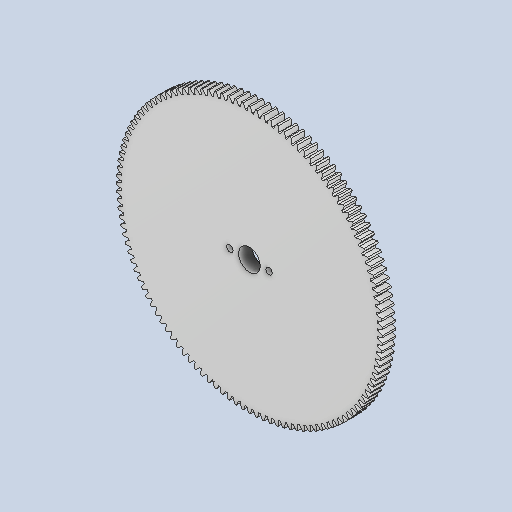
# Autodesk Inventor part: 平歯車1
Saved by Autodesk Inventor 2025.2 (Build 292293000, 293)
## iProperties
CustomPartVersion: 1
Created: 2025-01-13
Part Number: 平歯車1
Material: ABS プラスチック
Document SubType Name: Modeling
Designer: haruy
Categories: <?xml version="1.0" encoding="UTF-16"?> <MemberInstance><Categories><FamilyTemplate><FamilyTemplateParameter ValueType="xs:double" Id="1" ObjectReferenceKey="da_z" ObjectType="kUserParameterObject"/><FamilyTemplateParameter ValueType="xs:double" Id="2" ObjectReferenceKey="da_b" ObjectType="kUserParameterObject"/><FamilyTemplateParameter ValueType="xs:double" Id="3" ObjectReferenceKey="da_beta" ObjectType="kUserParameterObject"/><FamilyTemplateParameter ValueType="xs:double" Id="4" ObjectReferenceKey="da_da" ObjectType="kUserParameterObject"/><FamilyTemplateParameter ValueType="xs:double" Id="5" ObjectReferenceKey="da_aw" ObjectType="kUserParameterObject"/><FamilyTemplateParameter ValueType="xs:string" Id="6" ObjectReferenceKey="EAIAABAAAACIAQAAAAAAAIAAAAAAAAAA" ObjectType="83910656" SubObjectId="SurfaceGeometry"/></FamilyTemplate><ParamToTemplateMap><ParamToTemplate CategoryParameter="//CategoryParameter[@InternalName='046C89C9-8512-4d59-83FE-43B91F4F132A']" TemplateParameter="1"/><ParamToTemplate CategoryParameter="//CategoryParameter[@InternalName='2552DF32-E462-4b46-AEBF-C6C7768E72AC']" TemplateParameter="2"/><ParamToTemplate CategoryParameter="//CategoryParameter[@InternalName='C9EE641D-15FC-4fae-A226-E94C4372FDD7']" TemplateParameter="3"/><ParamToTemplate><ParamToTemplate CategoryParameter="//CategoryParameter[@InternalName='00B6519A-459B-49c7-AD84-2E56D39A5744']" ConstantValue="0.000000"/></ParamToTemplate><ParamToTemplate><ParamToTemplate CategoryParameter="//CategoryParameter[@InternalName='04B31F0E-C7A6-4894-AA32-9629BEFACF47']" ConstantValue="1.000000"/></ParamToTemplate><ParamToTemplate><ParamToTemplate CategoryParameter="//CategoryParameter[@InternalName='43CBEC2E-7847-49e7-A936-2F7889FCB2D9']" ConstantValue="0.250000"/></ParamToTemplate><ParamToTemplate><ParamToTemplate CategoryParameter="//CategoryParameter[@InternalName='B1EFC894-105D-4ebd-86BF-FA20ED196853']" ConstantValue="0.350000"/></ParamToTemplate><ParamToTemplate><ParamToTemplate CategoryParameter="//CategoryParameter[@InternalName='51175063-3D10-4879-93E8-6246FE8B403D']" ConstantValue="2060000000.000000"/></ParamToTemplate><ParamToTemplate><ParamToTemplate CategoryParameter="//CategoryParameter[@InternalName='A3A52E27-4454-46a9-B0BD-C932399B70AF']" ConstantValue="0.300000"/></ParamToTemplate><ParamToTemplate><ParamToTemplate CategoryParameter="//CategoryParameter[@InternalName='91B76062-C214-41d9-B1B9-14D2AB99603D']" ConstantValue="0.100000"/></ParamToTemplate><ParamToTemplate><ParamToTemplate CategoryParameter="//CategoryParameter[@InternalName='374E806E-8B8A-4dda-A9AA-1039D6500AD2']" ConstantValue="10.000000"/></ParamToTemplate><ParamToTemplate><ParamToTemplate CategoryParameter="//CategoryParameter[@InternalName='2D373A89-B862-43d6-8D0B-0CBF12AB9F6C']" ConstantValue="0.349066"/></ParamToTemplate><ParamToTemplate CategoryParameter="//CategoryParameter[@InternalName='37777632-D6A2-4fac-9D53-DB8ACD95C989']" TemplateParameter="4"/><ParamToTemplate CategoryParameter="//CategoryParameter[@InternalName='FD1017F1-B727-4f7e-9707-0F86F1FF9423']" TemplateParameter="5"/><ParamToTemplate><ParamToTemplate CategoryParameter="//CategoryParameter[@InternalName='9E1B4470-B2D3-4ff1-B813-535BB4CDF51A']" ConstantValue="3520000.000000"/></ParamToTemplate><ParamToTemplate><ParamToTemplate CategoryParameter="//CategoryParameter[@InternalName='F8452263-BFF6-458c-9FB1-07C4B99E95CD']" ConstantValue="11400000.000000"/></ParamToTemplate><ParamToTemplate><ParamToTemplate CategoryParameter="//CategoryParameter[@InternalName='3E3BB259-FD49-497f-8171-6EBC954A3479']" ConstantValue="2.000000"/></ParamToTemplate><ParamToTemplate CategoryParameter="//CategoryParameter[@InternalName='27C3BAF2-7550-4e4b-AE2C-0DB134B7D9B7']" TemplateParameter="6"/></ParamToTemplateMap><Category DisplayName="Gear" InternalName="DC85795E-93AB-48d5-8EEE-5A27447B64BD" Mnemonic="Gear"><CategoryParameter DisplayName="z" InternalName="046C89C9-8512-4d59-83FE-43B91F4F132A" Mnemonic="z"/><CategoryParameter DisplayName="b" InternalName="2552DF32-E462-4b46-AEBF-C6C7768E72AC" Mnemonic="b"/><CategoryParameter DisplayName="||b|" InternalName="C9EE641D-15FC-4fae-A226-E94C4372FDD7" Mnemonic="beta"/><CategoryParameter DisplayName="x" InternalName="00B6519A-459B-49c7-AD84-2E56D39A5744" Mnemonic="x"/><CategoryParameter DisplayName="a*" InternalName="04B31F0E-C7A6-4894-AA32-9629BEFACF47" Mnemonic="a"/><CategoryParameter DisplayName="c*" InternalName="43CBEC2E-7847-49e7-A936-2F7889FCB2D9" Mnemonic="c"/><CategoryParameter DisplayName="r|.f|*" InternalName="B1EFC894-105D-4ebd-86BF-FA20ED196853" Mnemonic="rf"/><CategoryParameter DisplayName="E" InternalName="51175063-3D10-4879-93E8-6246FE8B403D" Mnemonic="E"/><CategoryParameter DisplayName="||m|" InternalName="A3A52E27-4454-46a9-B0BD-C932399B70AF" Mnemonic="mi"/><Category DisplayName="SpurGear" InternalName="26C5A22E-A91E-4dfd-A3B3-23CCAFAE1764" Mnemonic="SpurGear"><CategoryParameter DisplayName="m" InternalName="91B76062-C214-41d9-B1B9-14D2AB99603D" Mnemonic="m"/><CategoryParameter DisplayName="P" InternalName="374E806E-8B8A-4dda-A9AA-1039D6500AD2" Mnemonic="PP"/><CategoryParameter DisplayName="||a|" InternalName="2D373A89-B862-43d6-8D0B-0CBF12AB9F6C" Mnemonic="alpha"/><CategoryParameter DisplayName="d|.a|" InternalName="37777632-D6A2-4fac-9D53-DB8ACD95C989" Mnemonic="da"/><CategoryParameter DisplayName="a|.w|" InternalName="FD1017F1-B727-4f7e-9707-0F86F1FF9423" Mnemonic="aw"/><CategoryParameter DisplayName="||s||.Flim|" InternalName="9E1B4470-B2D3-4ff1-B813-535BB4CDF51A" Mnemonic="sFlim"/><CategoryParameter DisplayName="||s||.Hlim|" InternalName="F8452263-BFF6-458c-9FB1-07C4B99E95CD" Mnemonic="sHlim"/><CategoryParameter DisplayName="タイプ" InternalName="3E3BB259-FD49-497f-8171-6EBC954A3479" Mnemonic="type"/><CategoryParameter DisplayName="PitchDiameter" InternalName="27C3BAF2-7550-4e4b-AE2C-0DB134B7D9B7" Mnemonic="IDS_PITCHDIAM"/></Category></Category></Categories></MemberInstance>
Density: 1.06 g/cm^3
Appearance: 滑らか - 白
Mass: 531.343 g
Surface Area: 271.257 cm^2
Volume: 67.687 cm^3
Author: haruy
Autodesk Inventor part; units mm, degrees
sketch "Sketch1" plane through (0, 0, 0) normal (0, 0, 1) x (1, 0, 0)
  circle A0 centre (0, 0) radius 61
  dimension "d0" = 122
  constraints: 1 centre point
  measures "d0" diameter of A0
extrude "Extrusion1" add sketch "Sketch1" along normal blind 6
ref_plane "Work Plane2" through (0, 0, 3) normal (0, 0, 1) x (1, 0, 0)
sketch "Sketch2" plane through (0, 0, 0) normal (0, 0, -1) x (-1, 0, 0)
  circle A0 centre (0, 0) radius 61 projected
  circle A1 centre (0, 0) radius 60
  dimension "d3" = 120
  constraints: 1 centre point, 1 coincident
  measures "d3" diameter of A1
surface extrude "ピッチ円直径" sketch "Sketch2" against normal through all shown no curves A1
ref_plane "Work Plane8" through (0, 0, 0) normal (0.9996573, 0.0261769, 0) x (0, 0, 1)
ref_plane "Work Plane9" through (0, 0, 0) normal (1, 0, 0) x (0, 1, 0)
spur gear teeth "平歯車" teeth 120 pitch diameter 120 tip diameter 122 root diameter 117.5 face width 6 start plane through (0, 0, 0) normal (0, 0, -1) x (-1, 0, 0)
sketch "スケッチ3" plane through (0, 0, 6) normal (0, 0, 1) x (1, 0, 0)
  circle A0 centre (0, 0) radius 5
  circle A1 centre (0, 0) radius 9
  circle A2 centre (-9, 0) radius 1.5
  circle A3 centre (9, 0) radius 1.5
  dimension "d50" = 18
  dimension "d49" = 10
  dimension "d51" = 3
  dimension "d54" = 360
  constraints: 3 centre point, 2 coincident, 1 horizontal alignment, 7 other
  measures "d49" diameter of A0
  measures "d51" diameter of A2
extrude "押し出し2" cut sketch "スケッチ3" against normal blind 10 contours A0 | A1 A3 | A1 A3 | A2 A1 | A1 A2
sketch "スケッチ4" plane through (0, 0, 6) normal (0, 0, 1) x (1, 0, 0)
  circle A0 centre (9, 0) radius 1.5 projected
  circle A1 centre (0, 0) radius 5 projected
  circle A2 centre (-9, 0) radius 1.5 projected
  arc A3 (-3.5911, 60.8942) -> (-4.226, 58.5978) centre (10.0352, 55.8907) ccw projected
  arc A4 (-4.226, 58.5978) -> (-4.9927, 58.5375) centre (0, 0) ccw projected
  arc A5 (-4.9927, 58.5375) -> (-5.979, 60.7063) centre (-18.6549, 53.6328) ccw projected
  arc A6 (-5.979, 60.7063) -> (-6.7732, 60.6228) centre (0, 0) ccw projected
  arc A7 (-6.7732, 60.6228) -> (-7.287, 58.2963) centre (7.0963, 56.3393) ccw projected
  arc A8 (-7.287, 58.2963) -> (-8.0495, 58.1959) centre (0, 0) ccw projected
  arc A9 (-8.0495, 58.1959) -> (-9.148, 60.3102) centre (-21.4362, 52.5829) ccw projected
  arc A10 (-9.148, 60.3102) -> (-9.9366, 60.1852) centre (0, 0) ccw projected
  arc A11 (-9.9366, 60.1852) -> (-10.328, 57.8351) centre (4.138, 56.6335) ccw projected
  arc A12 (-10.328, 57.8351) -> (-11.0842, 57.6949) centre (0, 0) ccw projected
  arc A13 (-11.0842, 57.6949) -> (-12.2918, 59.7487) centre (-24.1588, 51.389) ccw projected
  arc A14 (-12.2918, 59.7487) -> (-13.0729, 59.5827) centre (0, 0) ccw projected
  arc A15 (-13.0729, 59.5827) -> (-13.3407, 57.2153) centre (1.1684, 56.7725) ccw projected
  arc A16 (-13.3407, 57.2153) -> (-14.0885, 57.0357) centre (0, 0) ccw projected
  arc A17 (-14.0885, 57.0357) -> (-15.402, 59.0235) centre (-26.8152, 50.0542) ccw projected
  arc A18 (-15.402, 59.0235) -> (-16.1733, 58.8169) centre (0, 0) ccw projected
  arc A19 (-16.1733, 58.8169) -> (-16.3169, 56.4387) centre (-1.8044, 56.7558) ccw projected
  arc A20 (-16.3169, 56.4387) -> (-17.0542, 56.2202) centre (0, 0) ccw projected
  arc A21 (-17.0542, 56.2202) -> (-18.4699, 58.1366) centre (-29.3981, 48.5822) ccw projected
  arc A22 (-18.4699, 58.1366) -> (-19.2293, 57.8898) centre (0, 0) ccw projected
  arc A23 (-19.2293, 57.8898) -> (-19.2483, 55.5074) centre (-4.7723, 56.5836) ccw projected
  arc A24 (-19.2483, 55.5074) -> (-19.9732, 55.2506) centre (0, 0) ccw projected
  arc A25 (-19.9732, 55.2506) -> (-21.4873, 57.0903) centre (-31.9004, 46.977) ccw projected
  arc A26 (-21.4873, 57.0903) -> (-22.2327, 56.8041) centre (0, 0) ccw projected
  arc A27 (-22.2327, 56.8041) -> (-22.1269, 54.4239) centre (-7.7272, 56.2563) ccw projected
  arc A28 (-22.1269, 54.4239) -> (-22.8374, 54.1296) centre (0, 0) ccw projected
  arc A29 (-22.8374, 54.1296) -> (-24.4457, 55.8875) centre (-34.3153, 45.2431) ccw projected
  arc A30 (-24.4457, 55.8875) -> (-25.1751, 55.5627) centre (0, 0) ccw projected
  arc A31 (-25.1751, 55.5627) -> (-24.9449, 53.1913) centre (-10.6608, 55.7748) ccw projected
  arc A32 (-24.9449, 53.1913) -> (-25.639, 52.8602) centre (0, 0) ccw projected
  arc A33 (-25.639, 52.8602) -> (-27.3371, 54.5315) centre (-36.6361, 43.3852) ccw projected
  arc A34 (-27.3371, 54.5315) -> (-28.0486, 54.169) centre (0, 0) ccw projected
  arc A35 (-28.0486, 54.169) -> (-27.6946, 51.8129) centre (-13.5652, 55.1404) ccw projected
  arc A36 (-27.6946, 51.8129) -> (-28.3704, 51.4459) centre (0, 0) ccw projected
  arc A37 (-28.3704, 51.4459) -> (-30.1536, 53.026) centre (-38.8565, 41.4084) ccw projected
  arc A38 (-30.1536, 53.026) -> (-30.8451, 52.6268) centre (0, 0) ccw projected
  arc A39 (-30.8451, 52.6268) -> (-30.3683, 50.2924) centre (-16.4324, 54.3549) ccw projected
  arc A40 (-30.3683, 50.2924) -> (-31.024, 49.8906) centre (0, 0) ccw projected
  arc A41 (-31.024, 49.8906) -> (-32.8874, 51.3753) centre (-40.9704, 39.318) ccw projected
  arc A42 (-32.8874, 51.3753) -> (-33.5571, 50.9404) centre (0, 0) ccw projected
  arc A43 (-33.5571, 50.9404) -> (-32.9588, 48.6342) centre (-19.2546, 53.4204) ccw projected
  arc A44 (-32.9588, 48.6342) -> (-33.5925, 48.1986) centre (0, 0) ccw projected
  arc A45 (-33.5925, 48.1986) -> (-35.5311, 49.5836) centre (-42.972, 37.1199) ccw projected
  arc A46 (-35.5311, 49.5836) -> (-36.1771, 49.1143) centre (0, 0) ccw projected
  arc A47 (-36.1771, 49.1143) -> (-35.4589, 46.8426) centre (-22.0241, 52.3395) ccw projected
  arc A48 (-35.4589, 46.8426) -> (-36.069, 46.3744) centre (0, 0) ccw projected
  arc A49 (-36.069, 46.3744) -> (-38.0775, 47.6561) centre (-44.8558, 34.8201) ccw projected
  arc A50 (-38.0775, 47.6561) -> (-38.698, 47.1536) centre (0, 0) ccw projected
  arc A51 (-38.698, 47.1536) -> (-37.8619, 44.9226) centre (-24.7331, 51.1151) ccw projected
  arc A52 (-37.8619, 44.9226) -> (-38.4466, 44.4232) centre (0, 0) ccw projected
  arc A53 (-38.4466, 44.4232) -> (-40.5194, 45.598) centre (-46.6167, 32.4248) ccw projected
  arc A54 (-40.5194, 45.598) -> (-41.1128, 45.0637) centre (0, 0) ccw projected
  arc A55 (-41.1128, 45.0637) -> (-40.161, 42.8795) centre (-27.3744, 49.7506) ccw projected
  arc A56 (-40.161, 42.8795) -> (-40.7189, 42.3501) centre (0, 0) ccw projected
  arc A57 (-40.7189, 42.3501) -> (-42.8503, 43.4149) centre (-48.2498, 29.9406) ccw projected
  arc A58 (-42.8503, 43.4149) -> (-43.4149, 42.8503) centre (0, 0) ccw projected
  arc A59 (-43.4149, 42.8503) -> (-42.3501, 40.7189) centre (-29.9406, 48.2498) ccw projected
  arc A60 (-42.3501, 40.7189) -> (-42.8795, 40.161) centre (0, 0) ccw projected
  arc A61 (-42.8795, 40.161) -> (-45.0637, 41.1128) centre (-49.7506, 27.3744) ccw projected
  arc A62 (-45.0637, 41.1128) -> (-45.598, 40.5194) centre (0, 0) ccw projected
  arc A63 (-45.598, 40.5194) -> (-44.4232, 38.4466) centre (-32.4248, 46.6167) ccw projected
  arc A64 (-44.4232, 38.4466) -> (-44.9226, 37.8619) centre (0, 0) ccw projected
  arc A65 (-44.9226, 37.8619) -> (-47.1536, 38.698) centre (-51.1151, 24.7331) ccw projected
  arc A66 (-47.1536, 38.698) -> (-47.6561, 38.0775) centre (0, 0) ccw projected
  arc A67 (-47.6561, 38.0775) -> (-46.3744, 36.069) centre (-34.8201, 44.8558) ccw projected
  arc A68 (-46.3744, 36.069) -> (-46.8426, 35.4589) centre (0, 0) ccw projected
  arc A69 (-46.8426, 35.4589) -> (-49.1143, 36.1771) centre (-52.3395, 22.0241) ccw projected
  arc A70 (-49.1143, 36.1771) -> (-49.5836, 35.5311) centre (0, 0) ccw projected
  arc A71 (-49.5836, 35.5311) -> (-48.1986, 33.5925) centre (-37.1199, 42.972) ccw projected
  arc A72 (-48.1986, 33.5925) -> (-48.6342, 32.9588) centre (0, 0) ccw projected
  arc A73 (-48.6342, 32.9588) -> (-50.9404, 33.5571) centre (-53.4204, 19.2546) ccw projected
  arc A74 (-50.9404, 33.5571) -> (-51.3753, 32.8874) centre (0, 0) ccw projected
  arc A75 (-51.3753, 32.8874) -> (-49.8906, 31.024) centre (-39.318, 40.9704) ccw projected
  arc A76 (-49.8906, 31.024) -> (-50.2924, 30.3683) centre (0, 0) ccw projected
  arc A77 (-50.2924, 30.3683) -> (-52.6268, 30.8451) centre (-54.3549, 16.4324) ccw projected
  arc A78 (-52.6268, 30.8451) -> (-53.026, 30.1536) centre (0, 0) ccw projected
  arc A79 (-53.026, 30.1536) -> (-51.4459, 28.3704) centre (-41.4084, 38.8565) ccw projected
  arc A80 (-51.4459, 28.3704) -> (-51.8129, 27.6946) centre (0, 0) ccw projected
  arc A81 (-51.8129, 27.6946) -> (-54.169, 28.0486) centre (-55.1404, 13.5652) ccw projected
  arc A82 (-54.169, 28.0486) -> (-54.5315, 27.3371) centre (0, 0) ccw projected
  arc A83 (-54.5315, 27.3371) -> (-52.8602, 25.639) centre (-43.3852, 36.6361) ccw projected
  arc A84 (-52.8602, 25.639) -> (-53.1913, 24.9449) centre (0, 0) ccw projected
  arc A85 (-53.1913, 24.9449) -> (-55.5627, 25.1751) centre (-55.7748, 10.6608) ccw projected
  arc A86 (-55.5627, 25.1751) -> (-55.8875, 24.4457) centre (0, 0) ccw projected
  arc A87 (-55.8875, 24.4457) -> (-54.1296, 22.8374) centre (-45.2431, 34.3153) ccw projected
  arc A88 (-54.1296, 22.8374) -> (-54.4239, 22.1269) centre (0, 0) ccw projected
  arc A89 (-54.4239, 22.1269) -> (-56.8041, 22.2327) centre (-56.2563, 7.7272) ccw projected
  arc A90 (-56.8041, 22.2327) -> (-57.0903, 21.4873) centre (0, 0) ccw projected
  arc A91 (-57.0903, 21.4873) -> (-55.2506, 19.9732) centre (-46.977, 31.9004) ccw projected
  arc A92 (-55.2506, 19.9732) -> (-55.5074, 19.2483) centre (0, 0) ccw projected
  arc A93 (-55.5074, 19.2483) -> (-57.8898, 19.2293) centre (-56.5836, 4.7723) ccw projected
  arc A94 (-57.8898, 19.2293) -> (-58.1366, 18.4699) centre (0, 0) ccw projected
  arc A95 (-58.1366, 18.4699) -> (-56.2202, 17.0542) centre (-48.5822, 29.3981) ccw projected
  arc A96 (-56.2202, 17.0542) -> (-56.4387, 16.3169) centre (0, 0) ccw projected
  arc A97 (-56.4387, 16.3169) -> (-58.8169, 16.1733) centre (-56.7558, 1.8044) ccw projected
  arc A98 (-58.8169, 16.1733) -> (-59.0235, 15.402) centre (0, 0) ccw projected
  arc A99 (-59.0235, 15.402) -> (-57.0357, 14.0885) centre (-50.0542, 26.8152) ccw projected
  arc A100 (-57.0357, 14.0885) -> (-57.2153, 13.3407) centre (0, 0) ccw projected
  arc A101 (-57.2153, 13.3407) -> (-59.5827, 13.0729) centre (-56.7725, -1.1684) ccw projected
  arc A102 (-59.5827, 13.0729) -> (-59.7487, 12.2918) centre (0, 0) ccw projected
  arc A103 (-59.7487, 12.2918) -> (-57.6949, 11.0842) centre (-51.389, 24.1588) ccw projected
  arc A104 (-57.6949, 11.0842) -> (-57.8351, 10.328) centre (0, 0) ccw projected
  arc A105 (-57.8351, 10.328) -> (-60.1852, 9.9366) centre (-56.6335, -4.138) ccw projected
  arc A106 (-60.1852, 9.9366) -> (-60.3102, 9.148) centre (0, 0) ccw projected
  arc A107 (-60.3102, 9.148) -> (-58.1959, 8.0495) centre (-52.5829, 21.4362) ccw projected
  arc A108 (-58.1959, 8.0495) -> (-58.2963, 7.287) centre (0, 0) ccw projected
  arc A109 (-58.2963, 7.287) -> (-60.6228, 6.7732) centre (-56.3393, -7.0963) ccw projected
  arc A110 (-60.6228, 6.7732) -> (-60.7063, 5.979) centre (0, 0) ccw projected
  arc A111 (-60.7063, 5.979) -> (-58.5375, 4.9927) centre (-53.6328, 18.6549) ccw projected
  arc A112 (-58.5375, 4.9927) -> (-58.5978, 4.226) centre (0, 0) ccw projected
  arc A113 (-58.5978, 4.226) -> (-60.8942, 3.5911) centre (-55.8907, -10.0352) ccw projected
  arc A114 (-60.8942, 3.5911) -> (-60.936, 2.7937) centre (0, 0) ccw projected
  arc A115 (-60.936, 2.7937) -> (-58.7185, 1.9222) centre (-54.5356, 15.8224) ccw projected
  arc A116 (-58.7185, 1.9222) -> (-58.7387, 1.1535) centre (0, 0) ccw projected
  arc A117 (-58.7387, 1.1535) -> (-60.9987, 0.3992) centre (-55.2889, -12.9465) ccw projected
  arc A118 (-60.9987, 0.3992) -> (-60.9987, -0.3992) centre (0, 0) ccw projected
  arc A119 (-60.9987, -0.3992) -> (-58.7387, -1.1535) centre (-55.2889, 12.9465) ccw projected
  arc A120 (-58.7387, -1.1535) -> (-58.7185, -1.9222) centre (0, 0) ccw projected
  arc A121 (-58.7185, -1.9222) -> (-60.936, -2.7937) centre (-54.5356, -15.8224) ccw projected
  arc A122 (-60.936, -2.7937) -> (-60.8942, -3.5911) centre (0, 0) ccw projected
  arc A123 (-60.8942, -3.5911) -> (-58.5978, -4.226) centre (-55.8907, 10.0352) ccw projected
  arc A124 (-58.5978, -4.226) -> (-58.5375, -4.9927) centre (0, 0) ccw projected
  arc A125 (-58.5375, -4.9927) -> (-60.7063, -5.979) centre (-53.6328, -18.6549) ccw projected
  arc A126 (-60.7063, -5.979) -> (-60.6228, -6.7732) centre (0, 0) ccw projected
  arc A127 (-60.6228, -6.7732) -> (-58.2963, -7.287) centre (-56.3393, 7.0963) ccw projected
  arc A128 (-58.2963, -7.287) -> (-58.1959, -8.0495) centre (0, 0) ccw projected
  arc A129 (-58.1959, -8.0495) -> (-60.3102, -9.148) centre (-52.5829, -21.4362) ccw projected
  arc A130 (-60.3102, -9.148) -> (-60.1852, -9.9366) centre (0, 0) ccw projected
  arc A131 (-60.1852, -9.9366) -> (-57.8351, -10.328) centre (-56.6335, 4.138) ccw projected
  arc A132 (-57.8351, -10.328) -> (-57.6949, -11.0842) centre (0, 0) ccw projected
  arc A133 (-57.6949, -11.0842) -> (-59.7487, -12.2918) centre (-51.389, -24.1588) ccw projected
  arc A134 (-59.7487, -12.2918) -> (-59.5827, -13.0729) centre (0, 0) ccw projected
  arc A135 (-59.5827, -13.0729) -> (-57.2153, -13.3407) centre (-56.7725, 1.1684) ccw projected
  arc A136 (-57.2153, -13.3407) -> (-57.0357, -14.0885) centre (0, 0) ccw projected
  arc A137 (-57.0357, -14.0885) -> (-59.0235, -15.402) centre (-50.0542, -26.8152) ccw projected
  arc A138 (-59.0235, -15.402) -> (-58.8169, -16.1733) centre (0, 0) ccw projected
  arc A139 (-58.8169, -16.1733) -> (-56.4387, -16.3169) centre (-56.7558, -1.8044) ccw projected
  arc A140 (-56.4387, -16.3169) -> (-56.2202, -17.0542) centre (0, 0) ccw projected
  arc A141 (-56.2202, -17.0542) -> (-58.1366, -18.4699) centre (-48.5822, -29.3981) ccw projected
  arc A142 (-58.1366, -18.4699) -> (-57.8898, -19.2293) centre (0, 0) ccw projected
  arc A143 (-57.8898, -19.2293) -> (-55.5074, -19.2483) centre (-56.5836, -4.7723) ccw projected
  arc A144 (-55.5074, -19.2483) -> (-55.2506, -19.9732) centre (0, 0) ccw projected
  arc A145 (-55.2506, -19.9732) -> (-57.0903, -21.4873) centre (-46.977, -31.9004) ccw projected
  arc A146 (-57.0903, -21.4873) -> (-56.8041, -22.2327) centre (0, 0) ccw projected
  arc A147 (-56.8041, -22.2327) -> (-54.4239, -22.1269) centre (-56.2563, -7.7272) ccw projected
  arc A148 (-54.4239, -22.1269) -> (-54.1296, -22.8374) centre (0, 0) ccw projected
  arc A149 (-54.1296, -22.8374) -> (-55.8875, -24.4457) centre (-45.2431, -34.3153) ccw projected
  arc A150 (-55.8875, -24.4457) -> (-55.5627, -25.1751) centre (0, 0) ccw projected
  arc A151 (-55.5627, -25.1751) -> (-53.1913, -24.9449) centre (-55.7748, -10.6608) ccw projected
  arc A152 (-53.1913, -24.9449) -> (-52.8602, -25.639) centre (0, 0) ccw projected
  arc A153 (-52.8602, -25.639) -> (-54.5315, -27.3371) centre (-43.3852, -36.6361) ccw projected
  arc A154 (-54.5315, -27.3371) -> (-54.169, -28.0486) centre (0, 0) ccw projected
  arc A155 (-54.169, -28.0486) -> (-51.8129, -27.6946) centre (-55.1404, -13.5652) ccw projected
  arc A156 (-51.8129, -27.6946) -> (-51.4459, -28.3704) centre (0, 0) ccw projected
  arc A157 (-51.4459, -28.3704) -> (-53.026, -30.1536) centre (-41.4084, -38.8565) ccw projected
  arc A158 (-53.026, -30.1536) -> (-52.6268, -30.8451) centre (0, 0) ccw projected
  arc A159 (-52.6268, -30.8451) -> (-50.2924, -30.3683) centre (-54.3549, -16.4324) ccw projected
  arc A160 (-50.2924, -30.3683) -> (-49.8906, -31.024) centre (0, 0) ccw projected
  arc A161 (-49.8906, -31.024) -> (-51.3753, -32.8874) centre (-39.318, -40.9704) ccw projected
  arc A162 (-51.3753, -32.8874) -> (-50.9404, -33.5571) centre (0, 0) ccw projected
  arc A163 (-50.9404, -33.5571) -> (-48.6342, -32.9588) centre (-53.4204, -19.2546) ccw projected
  arc A164 (-48.6342, -32.9588) -> (-48.1986, -33.5925) centre (0, 0) ccw projected
  arc A165 (-48.1986, -33.5925) -> (-49.5836, -35.5311) centre (-37.1199, -42.972) ccw projected
  arc A166 (-49.5836, -35.5311) -> (-49.1143, -36.1771) centre (0, 0) ccw projected
  arc A167 (-49.1143, -36.1771) -> (-46.8426, -35.4589) centre (-52.3395, -22.0241) ccw projected
  arc A168 (-46.8426, -35.4589) -> (-46.3744, -36.069) centre (0, 0) ccw projected
  arc A169 (-46.3744, -36.069) -> (-47.6561, -38.0775) centre (-34.8201, -44.8558) ccw projected
  arc A170 (-47.6561, -38.0775) -> (-47.1536, -38.698) centre (0, 0) ccw projected
  arc A171 (-47.1536, -38.698) -> (-44.9226, -37.8619) centre (-51.1151, -24.7331) ccw projected
  arc A172 (-44.9226, -37.8619) -> (-44.4232, -38.4466) centre (0, 0) ccw projected
  arc A173 (-44.4232, -38.4466) -> (-45.598, -40.5194) centre (-32.4248, -46.6167) ccw projected
  arc A174 (-45.598, -40.5194) -> (-45.0637, -41.1128) centre (0, 0) ccw projected
  arc A175 (-45.0637, -41.1128) -> (-42.8795, -40.161) centre (-49.7506, -27.3744) ccw projected
  arc A176 (-42.8795, -40.161) -> (-42.3501, -40.7189) centre (0, 0) ccw projected
  arc A177 (-42.3501, -40.7189) -> (-43.4149, -42.8503) centre (-29.9406, -48.2498) ccw projected
  arc A178 (-43.4149, -42.8503) -> (-42.8503, -43.4149) centre (0, 0) ccw projected
  arc A179 (-42.8503, -43.4149) -> (-40.7189, -42.3501) centre (-48.2498, -29.9406) ccw projected
  arc A180 (-40.7189, -42.3501) -> (-40.161, -42.8795) centre (0, 0) ccw projected
  arc A181 (-40.161, -42.8795) -> (-41.1128, -45.0637) centre (-27.3744, -49.7506) ccw projected
  arc A182 (-41.1128, -45.0637) -> (-40.5194, -45.598) centre (0, 0) ccw projected
  arc A183 (-40.5194, -45.598) -> (-38.4466, -44.4232) centre (-46.6167, -32.4248) ccw projected
  arc A184 (-38.4466, -44.4232) -> (-37.8619, -44.9226) centre (0, 0) ccw projected
  arc A185 (-37.8619, -44.9226) -> (-38.698, -47.1536) centre (-24.7331, -51.1151) ccw projected
  arc A186 (-38.698, -47.1536) -> (-38.0775, -47.6561) centre (0, 0) ccw projected
  arc A187 (-38.0775, -47.6561) -> (-36.069, -46.3744) centre (-44.8558, -34.8201) ccw projected
  arc A188 (-36.069, -46.3744) -> (-35.4589, -46.8426) centre (0, 0) ccw projected
  arc A189 (-35.4589, -46.8426) -> (-36.1771, -49.1143) centre (-22.0241, -52.3395) ccw projected
  arc A190 (-36.1771, -49.1143) -> (-35.5311, -49.5836) centre (0, 0) ccw projected
  arc A191 (-35.5311, -49.5836) -> (-33.5925, -48.1986) centre (-42.972, -37.1199) ccw projected
  arc A192 (-33.5925, -48.1986) -> (-32.9588, -48.6342) centre (0, 0) ccw projected
  arc A193 (-32.9588, -48.6342) -> (-33.5571, -50.9404) centre (-19.2546, -53.4204) ccw projected
  arc A194 (-33.5571, -50.9404) -> (-32.8874, -51.3753) centre (0, 0) ccw projected
  arc A195 (-32.8874, -51.3753) -> (-31.024, -49.8906) centre (-40.9704, -39.318) ccw projected
  arc A196 (-31.024, -49.8906) -> (-30.3683, -50.2924) centre (0, 0) ccw projected
  arc A197 (-30.3683, -50.2924) -> (-30.8451, -52.6268) centre (-16.4324, -54.3549) ccw projected
  arc A198 (-30.8451, -52.6268) -> (-30.1536, -53.026) centre (0, 0) ccw projected
  arc A199 (-30.1536, -53.026) -> (-28.3704, -51.4459) centre (-38.8565, -41.4084) ccw projected
  arc A200 (-28.3704, -51.4459) -> (-27.6946, -51.8129) centre (0, 0) ccw projected
  arc A201 (-27.6946, -51.8129) -> (-28.0486, -54.169) centre (-13.5652, -55.1404) ccw projected
  arc A202 (-28.0486, -54.169) -> (-27.3371, -54.5315) centre (0, 0) ccw projected
  arc A203 (-27.3371, -54.5315) -> (-25.639, -52.8602) centre (-36.6361, -43.3852) ccw projected
  arc A204 (-25.639, -52.8602) -> (-24.9449, -53.1913) centre (0, 0) ccw projected
  arc A205 (-24.9449, -53.1913) -> (-25.1751, -55.5627) centre (-10.6608, -55.7748) ccw projected
  arc A206 (-25.1751, -55.5627) -> (-24.4457, -55.8875) centre (0, 0) ccw projected
  arc A207 (-24.4457, -55.8875) -> (-22.8374, -54.1296) centre (-34.3153, -45.2431) ccw projected
  arc A208 (-22.8374, -54.1296) -> (-22.1269, -54.4239) centre (0, 0) ccw projected
  arc A209 (-22.1269, -54.4239) -> (-22.2327, -56.8041) centre (-7.7272, -56.2563) ccw projected
  arc A210 (-22.2327, -56.8041) -> (-21.4873, -57.0903) centre (0, 0) ccw projected
  arc A211 (-21.4873, -57.0903) -> (-19.9732, -55.2506) centre (-31.9004, -46.977) ccw projected
  arc A212 (-19.9732, -55.2506) -> (-19.2483, -55.5074) centre (0, 0) ccw projected
  arc A213 (-19.2483, -55.5074) -> (-19.2293, -57.8898) centre (-4.7723, -56.5836) ccw projected
  arc A214 (-19.2293, -57.8898) -> (-18.4699, -58.1366) centre (0, 0) ccw projected
  arc A215 (-18.4699, -58.1366) -> (-17.0542, -56.2202) centre (-29.3981, -48.5822) ccw projected
  arc A216 (-17.0542, -56.2202) -> (-16.3169, -56.4387) centre (0, 0) ccw projected
  arc A217 (-16.3169, -56.4387) -> (-16.1733, -58.8169) centre (-1.8044, -56.7558) ccw projected
  arc A218 (-16.1733, -58.8169) -> (-15.402, -59.0235) centre (0, 0) ccw projected
  arc A219 (-15.402, -59.0235) -> (-14.0885, -57.0357) centre (-26.8152, -50.0542) ccw projected
  arc A220 (-14.0885, -57.0357) -> (-13.3407, -57.2153) centre (0, 0) ccw projected
  arc A221 (-13.3407, -57.2153) -> (-13.0729, -59.5827) centre (1.1684, -56.7725) ccw projected
  arc A222 (-13.0729, -59.5827) -> (-12.2918, -59.7487) centre (0, 0) ccw projected
  arc A223 (-12.2918, -59.7487) -> (-11.0842, -57.6949) centre (-24.1588, -51.389) ccw projected
  arc A224 (-11.0842, -57.6949) -> (-10.328, -57.8351) centre (0, 0) ccw projected
  arc A225 (-10.328, -57.8351) -> (-9.9366, -60.1852) centre (4.138, -56.6335) ccw projected
  arc A226 (-9.9366, -60.1852) -> (-9.148, -60.3102) centre (0, 0) ccw projected
  arc A227 (-9.148, -60.3102) -> (-8.0495, -58.1959) centre (-21.4362, -52.5829) ccw projected
  arc A228 (-8.0495, -58.1959) -> (-7.287, -58.2963) centre (0, 0) ccw projected
  arc A229 (-7.287, -58.2963) -> (-6.7732, -60.6228) centre (7.0963, -56.3393) ccw projected
  arc A230 (-6.7732, -60.6228) -> (-5.979, -60.7063) centre (0, 0) ccw projected
  arc A231 (-5.979, -60.7063) -> (-4.9927, -58.5375) centre (-18.6549, -53.6328) ccw projected
  arc A232 (-4.9927, -58.5375) -> (-4.226, -58.5978) centre (0, 0) ccw projected
  arc A233 (-4.226, -58.5978) -> (-3.5911, -60.8942) centre (10.0352, -55.8907) ccw projected
  arc A234 (-3.5911, -60.8942) -> (-2.7937, -60.936) centre (0, 0) ccw projected
  arc A235 (-2.7937, -60.936) -> (-1.9222, -58.7185) centre (-15.8224, -54.5356) ccw projected
  arc A236 (-1.9222, -58.7185) -> (-1.1535, -58.7387) centre (0, 0) ccw projected
  arc A237 (-1.1535, -58.7387) -> (-0.3992, -60.9987) centre (12.9465, -55.2889) ccw projected
  arc A238 (-0.3992, -60.9987) -> (0.3992, -60.9987) centre (0, 0) ccw projected
  arc A239 (0.3992, -60.9987) -> (1.1535, -58.7387) centre (-12.9465, -55.2889) ccw projected
  arc A240 (1.1535, -58.7387) -> (1.9222, -58.7185) centre (0, 0) ccw projected
  arc A241 (1.9222, -58.7185) -> (2.7937, -60.936) centre (15.8224, -54.5356) ccw projected
  arc A242 (2.7937, -60.936) -> (3.5911, -60.8942) centre (0, 0) ccw projected
  arc A243 (3.5911, -60.8942) -> (4.226, -58.5978) centre (-10.0352, -55.8907) ccw projected
  arc A244 (4.226, -58.5978) -> (4.9927, -58.5375) centre (0, 0) ccw projected
  arc A245 (4.9927, -58.5375) -> (5.979, -60.7063) centre (18.6549, -53.6328) ccw projected
  arc A246 (5.979, -60.7063) -> (6.7732, -60.6228) centre (0, 0) ccw projected
  arc A247 (6.7732, -60.6228) -> (7.287, -58.2963) centre (-7.0963, -56.3393) ccw projected
  arc A248 (7.287, -58.2963) -> (8.0495, -58.1959) centre (0, 0) ccw projected
  arc A249 (8.0495, -58.1959) -> (9.148, -60.3102) centre (21.4362, -52.5829) ccw projected
  arc A250 (9.148, -60.3102) -> (9.9366, -60.1852) centre (0, 0) ccw projected
  arc A251 (9.9366, -60.1852) -> (10.328, -57.8351) centre (-4.138, -56.6335) ccw projected
  arc A252 (10.328, -57.8351) -> (11.0842, -57.6949) centre (0, 0) ccw projected
  arc A253 (11.0842, -57.6949) -> (12.2918, -59.7487) centre (24.1588, -51.389) ccw projected
  arc A254 (12.2918, -59.7487) -> (13.0729, -59.5827) centre (0, 0) ccw projected
  arc A255 (13.0729, -59.5827) -> (13.3407, -57.2153) centre (-1.1684, -56.7725) ccw projected
  arc A256 (13.3407, -57.2153) -> (14.0885, -57.0357) centre (0, 0) ccw projected
  arc A257 (14.0885, -57.0357) -> (15.402, -59.0235) centre (26.8152, -50.0542) ccw projected
  arc A258 (15.402, -59.0235) -> (16.1733, -58.8169) centre (0, 0) ccw projected
  arc A259 (16.1733, -58.8169) -> (16.3169, -56.4387) centre (1.8044, -56.7558) ccw projected
  arc A260 (16.3169, -56.4387) -> (17.0542, -56.2202) centre (0, 0) ccw projected
  arc A261 (17.0542, -56.2202) -> (18.4699, -58.1366) centre (29.3981, -48.5822) ccw projected
  arc A262 (18.4699, -58.1366) -> (19.2293, -57.8898) centre (0, 0) ccw projected
  arc A263 (19.2293, -57.8898) -> (19.2483, -55.5074) centre (4.7723, -56.5836) ccw projected
  arc A264 (19.2483, -55.5074) -> (19.9732, -55.2506) centre (0, 0) ccw projected
  arc A265 (19.9732, -55.2506) -> (21.4873, -57.0903) centre (31.9004, -46.977) ccw projected
  arc A266 (21.4873, -57.0903) -> (22.2327, -56.8041) centre (0, 0) ccw projected
  arc A267 (22.2327, -56.8041) -> (22.1269, -54.4239) centre (7.7272, -56.2563) ccw projected
  arc A268 (22.1269, -54.4239) -> (22.8374, -54.1296) centre (0, 0) ccw projected
  arc A269 (22.8374, -54.1296) -> (24.4457, -55.8875) centre (34.3153, -45.2431) ccw projected
  arc A270 (24.4457, -55.8875) -> (25.1751, -55.5627) centre (0, 0) ccw projected
  arc A271 (25.1751, -55.5627) -> (24.9449, -53.1913) centre (10.6608, -55.7748) ccw projected
  arc A272 (24.9449, -53.1913) -> (25.639, -52.8602) centre (0, 0) ccw projected
  arc A273 (25.639, -52.8602) -> (27.3371, -54.5315) centre (36.6361, -43.3852) ccw projected
  arc A274 (27.3371, -54.5315) -> (28.0486, -54.169) centre (0, 0) ccw projected
  arc A275 (28.0486, -54.169) -> (27.6946, -51.8129) centre (13.5652, -55.1404) ccw projected
  arc A276 (27.6946, -51.8129) -> (28.3704, -51.4459) centre (0, 0) ccw projected
  arc A277 (28.3704, -51.4459) -> (30.1536, -53.026) centre (38.8565, -41.4084) ccw projected
  arc A278 (30.1536, -53.026) -> (30.8451, -52.6268) centre (0, 0) ccw projected
  arc A279 (30.8451, -52.6268) -> (30.3683, -50.2924) centre (16.4324, -54.3549) ccw projected
  arc A280 (30.3683, -50.2924) -> (31.024, -49.8906) centre (0, 0) ccw projected
  arc A281 (31.024, -49.8906) -> (32.8874, -51.3753) centre (40.9704, -39.318) ccw projected
  arc A282 (32.8874, -51.3753) -> (33.5571, -50.9404) centre (0, 0) ccw projected
  arc A283 (33.5571, -50.9404) -> (32.9588, -48.6342) centre (19.2546, -53.4204) ccw projected
  arc A284 (32.9588, -48.6342) -> (33.5925, -48.1986) centre (0, 0) ccw projected
  arc A285 (33.5925, -48.1986) -> (35.5311, -49.5836) centre (42.972, -37.1199) ccw projected
  arc A286 (35.5311, -49.5836) -> (36.1771, -49.1143) centre (0, 0) ccw projected
  arc A287 (36.1771, -49.1143) -> (35.4589, -46.8426) centre (22.0241, -52.3395) ccw projected
  arc A288 (35.4589, -46.8426) -> (36.069, -46.3744) centre (0, 0) ccw projected
  arc A289 (36.069, -46.3744) -> (38.0775, -47.6561) centre (44.8558, -34.8201) ccw projected
  arc A290 (38.0775, -47.6561) -> (38.698, -47.1536) centre (0, 0) ccw projected
  arc A291 (38.698, -47.1536) -> (37.8619, -44.9226) centre (24.7331, -51.1151) ccw projected
  arc A292 (37.8619, -44.9226) -> (38.4466, -44.4232) centre (0, 0) ccw projected
  arc A293 (38.4466, -44.4232) -> (40.5194, -45.598) centre (46.6167, -32.4248) ccw projected
  arc A294 (40.5194, -45.598) -> (41.1128, -45.0637) centre (0, 0) ccw projected
  arc A295 (41.1128, -45.0637) -> (40.161, -42.8795) centre (27.3744, -49.7506) ccw projected
  arc A296 (40.161, -42.8795) -> (40.7189, -42.3501) centre (0, 0) ccw projected
  arc A297 (40.7189, -42.3501) -> (42.8503, -43.4149) centre (48.2498, -29.9406) ccw projected
  arc A298 (42.8503, -43.4149) -> (43.4149, -42.8503) centre (0, 0) ccw projected
  arc A299 (43.4149, -42.8503) -> (42.3501, -40.7189) centre (29.9406, -48.2498) ccw projected
  arc A300 (42.3501, -40.7189) -> (42.8795, -40.161) centre (0, 0) ccw projected
  arc A301 (42.8795, -40.161) -> (45.0637, -41.1128) centre (49.7506, -27.3744) ccw projected
  arc A302 (45.0637, -41.1128) -> (45.598, -40.5194) centre (0, 0) ccw projected
  arc A303 (45.598, -40.5194) -> (44.4232, -38.4466) centre (32.4248, -46.6167) ccw projected
  arc A304 (44.4232, -38.4466) -> (44.9226, -37.8619) centre (0, 0) ccw projected
  arc A305 (44.9226, -37.8619) -> (47.1536, -38.698) centre (51.1151, -24.7331) ccw projected
  arc A306 (47.1536, -38.698) -> (47.6561, -38.0775) centre (0, 0) ccw projected
  arc A307 (47.6561, -38.0775) -> (46.3744, -36.069) centre (34.8201, -44.8558) ccw projected
  arc A308 (46.3744, -36.069) -> (46.8426, -35.4589) centre (0, 0) ccw projected
  arc A309 (46.8426, -35.4589) -> (49.1143, -36.1771) centre (52.3395, -22.0241) ccw projected
  arc A310 (49.1143, -36.1771) -> (49.5836, -35.5311) centre (0, 0) ccw projected
  arc A311 (49.5836, -35.5311) -> (48.1986, -33.5925) centre (37.1199, -42.972) ccw projected
  arc A312 (48.1986, -33.5925) -> (48.6342, -32.9588) centre (0, 0) ccw projected
  arc A313 (48.6342, -32.9588) -> (50.9404, -33.5571) centre (53.4204, -19.2546) ccw projected
  arc A314 (50.9404, -33.5571) -> (51.3753, -32.8874) centre (0, 0) ccw projected
  arc A315 (51.3753, -32.8874) -> (49.8906, -31.024) centre (39.318, -40.9704) ccw projected
  arc A316 (49.8906, -31.024) -> (50.2924, -30.3683) centre (0, 0) ccw projected
  arc A317 (50.2924, -30.3683) -> (52.6268, -30.8451) centre (54.3549, -16.4324) ccw projected
  arc A318 (52.6268, -30.8451) -> (53.026, -30.1536) centre (0, 0) ccw projected
  arc A319 (53.026, -30.1536) -> (51.4459, -28.3704) centre (41.4084, -38.8565) ccw projected
  arc A320 (51.4459, -28.3704) -> (51.8129, -27.6946) centre (0, 0) ccw projected
  arc A321 (51.8129, -27.6946) -> (54.169, -28.0486) centre (55.1404, -13.5652) ccw projected
  arc A322 (54.169, -28.0486) -> (54.5315, -27.3371) centre (0, 0) ccw projected
  arc A323 (54.5315, -27.3371) -> (52.8602, -25.639) centre (43.3852, -36.6361) ccw projected
  arc A324 (52.8602, -25.639) -> (53.1913, -24.9449) centre (0, 0) ccw projected
  arc A325 (53.1913, -24.9449) -> (55.5627, -25.1751) centre (55.7748, -10.6608) ccw projected
  arc A326 (55.5627, -25.1751) -> (55.8875, -24.4457) centre (0, 0) ccw projected
  arc A327 (55.8875, -24.4457) -> (54.1296, -22.8374) centre (45.2431, -34.3153) ccw projected
  arc A328 (54.1296, -22.8374) -> (54.4239, -22.1269) centre (0, 0) ccw projected
  arc A329 (54.4239, -22.1269) -> (56.8041, -22.2327) centre (56.2563, -7.7272) ccw projected
  arc A330 (56.8041, -22.2327) -> (57.0903, -21.4873) centre (0, 0) ccw projected
  arc A331 (57.0903, -21.4873) -> (55.2506, -19.9732) centre (46.977, -31.9004) ccw projected
  arc A332 (55.2506, -19.9732) -> (55.5074, -19.2483) centre (0, 0) ccw projected
  arc A333 (55.5074, -19.2483) -> (57.8898, -19.2293) centre (56.5836, -4.7723) ccw projected
  arc A334 (57.8898, -19.2293) -> (58.1366, -18.4699) centre (0, 0) ccw projected
  arc A335 (58.1366, -18.4699) -> (56.2202, -17.0542) centre (48.5822, -29.3981) ccw projected
  arc A336 (56.2202, -17.0542) -> (56.4387, -16.3169) centre (0, 0) ccw projected
  arc A337 (56.4387, -16.3169) -> (58.8169, -16.1733) centre (56.7558, -1.8044) ccw projected
  arc A338 (58.8169, -16.1733) -> (59.0235, -15.402) centre (0, 0) ccw projected
  arc A339 (59.0235, -15.402) -> (57.0357, -14.0885) centre (50.0542, -26.8152) ccw projected
  arc A340 (57.0357, -14.0885) -> (57.2153, -13.3407) centre (0, 0) ccw projected
  arc A341 (57.2153, -13.3407) -> (59.5827, -13.0729) centre (56.7725, 1.1684) ccw projected
  arc A342 (59.5827, -13.0729) -> (59.7487, -12.2918) centre (0, 0) ccw projected
  arc A343 (59.7487, -12.2918) -> (57.6949, -11.0842) centre (51.389, -24.1588) ccw projected
  arc A344 (57.6949, -11.0842) -> (57.8351, -10.328) centre (0, 0) ccw projected
  arc A345 (57.8351, -10.328) -> (60.1852, -9.9366) centre (56.6335, 4.138) ccw projected
  arc A346 (60.1852, -9.9366) -> (60.3102, -9.148) centre (0, 0) ccw projected
  arc A347 (60.3102, -9.148) -> (58.1959, -8.0495) centre (52.5829, -21.4362) ccw projected
  arc A348 (58.1959, -8.0495) -> (58.2963, -7.287) centre (0, 0) ccw projected
  arc A349 (58.2963, -7.287) -> (60.6228, -6.7732) centre (56.3393, 7.0963) ccw projected
  arc A350 (60.6228, -6.7732) -> (60.7063, -5.979) centre (0, 0) ccw projected
  arc A351 (60.7063, -5.979) -> (58.5375, -4.9927) centre (53.6328, -18.6549) ccw projected
  arc A352 (58.5375, -4.9927) -> (58.5978, -4.226) centre (0, 0) ccw projected
  arc A353 (58.5978, -4.226) -> (60.8942, -3.5911) centre (55.8907, 10.0352) ccw projected
  arc A354 (60.8942, -3.5911) -> (60.936, -2.7937) centre (0, 0) ccw projected
  arc A355 (60.936, -2.7937) -> (58.7185, -1.9222) centre (54.5356, -15.8224) ccw projected
  arc A356 (58.7185, -1.9222) -> (58.7387, -1.1535) centre (0, 0) ccw projected
  arc A357 (58.7387, -1.1535) -> (60.9987, -0.3992) centre (55.2889, 12.9465) ccw projected
  arc A358 (60.9987, -0.3992) -> (60.9987, 0.3992) centre (0, 0) ccw projected
  arc A359 (60.9987, 0.3992) -> (58.7387, 1.1535) centre (55.2889, -12.9465) ccw projected
  arc A360 (58.7387, 1.1535) -> (58.7185, 1.9222) centre (0, 0) ccw projected
  arc A361 (58.7185, 1.9222) -> (60.936, 2.7937) centre (54.5356, 15.8224) ccw projected
  arc A362 (60.936, 2.7937) -> (60.8942, 3.5911) centre (0, 0) ccw projected
  arc A363 (60.8942, 3.5911) -> (58.5978, 4.226) centre (55.8907, -10.0352) ccw projected
  arc A364 (58.5978, 4.226) -> (58.5375, 4.9927) centre (0, 0) ccw projected
  arc A365 (58.5375, 4.9927) -> (60.7063, 5.979) centre (53.6328, 18.6549) ccw projected
  arc A366 (60.7063, 5.979) -> (60.6228, 6.7732) centre (0, 0) ccw projected
  arc A367 (60.6228, 6.7732) -> (58.2963, 7.287) centre (56.3393, -7.0963) ccw projected
  arc A368 (58.2963, 7.287) -> (58.1959, 8.0495) centre (0, 0) ccw projected
  arc A369 (58.1959, 8.0495) -> (60.3102, 9.148) centre (52.5829, 21.4362) ccw projected
  arc A370 (60.3102, 9.148) -> (60.1852, 9.9366) centre (0, 0) ccw projected
  arc A371 (60.1852, 9.9366) -> (57.8351, 10.328) centre (56.6335, -4.138) ccw projected
  arc A372 (57.8351, 10.328) -> (57.6949, 11.0842) centre (0, 0) ccw projected
  arc A373 (57.6949, 11.0842) -> (59.7487, 12.2918) centre (51.389, 24.1588) ccw projected
  arc A374 (59.7487, 12.2918) -> (59.5827, 13.0729) centre (0, 0) ccw projected
  arc A375 (59.5827, 13.0729) -> (57.2153, 13.3407) centre (56.7725, -1.1684) ccw projected
  arc A376 (57.2153, 13.3407) -> (57.0357, 14.0885) centre (0, 0) ccw projected
  arc A377 (57.0357, 14.0885) -> (59.0235, 15.402) centre (50.0542, 26.8152) ccw projected
  arc A378 (59.0235, 15.402) -> (58.8169, 16.1733) centre (0, 0) ccw projected
  arc A379 (58.8169, 16.1733) -> (56.4387, 16.3169) centre (56.7558, 1.8044) ccw projected
  arc A380 (56.4387, 16.3169) -> (56.2202, 17.0542) centre (0, 0) ccw projected
  arc A381 (56.2202, 17.0542) -> (58.1366, 18.4699) centre (48.5822, 29.3981) ccw projected
  arc A382 (58.1366, 18.4699) -> (57.8898, 19.2293) centre (0, 0) ccw projected
  arc A383 (57.8898, 19.2293) -> (55.5074, 19.2483) centre (56.5836, 4.7723) ccw projected
  arc A384 (55.5074, 19.2483) -> (55.2506, 19.9732) centre (0, 0) ccw projected
  arc A385 (55.2506, 19.9732) -> (57.0903, 21.4873) centre (46.977, 31.9004) ccw projected
  arc A386 (57.0903, 21.4873) -> (56.8041, 22.2327) centre (0, 0) ccw projected
  arc A387 (56.8041, 22.2327) -> (54.4239, 22.1269) centre (56.2563, 7.7272) ccw projected
  arc A388 (54.4239, 22.1269) -> (54.1296, 22.8374) centre (0, 0) ccw projected
  arc A389 (54.1296, 22.8374) -> (55.8875, 24.4457) centre (45.2431, 34.3153) ccw projected
  arc A390 (55.8875, 24.4457) -> (55.5627, 25.1751) centre (0, 0) ccw projected
  arc A391 (55.5627, 25.1751) -> (53.1913, 24.9449) centre (55.7748, 10.6608) ccw projected
  arc A392 (53.1913, 24.9449) -> (52.8602, 25.639) centre (0, 0) ccw projected
  arc A393 (52.8602, 25.639) -> (54.5315, 27.3371) centre (43.3852, 36.6361) ccw projected
  arc A394 (54.5315, 27.3371) -> (54.169, 28.0486) centre (0, 0) ccw projected
  arc A395 (54.169, 28.0486) -> (51.8129, 27.6946) centre (55.1404, 13.5652) ccw projected
  arc A396 (51.8129, 27.6946) -> (51.4459, 28.3704) centre (0, 0) ccw projected
  arc A397 (51.4459, 28.3704) -> (53.026, 30.1536) centre (41.4084, 38.8565) ccw projected
  arc A398 (53.026, 30.1536) -> (52.6268, 30.8451) centre (0, 0) ccw projected
  arc A399 (52.6268, 30.8451) -> (50.2924, 30.3683) centre (54.3549, 16.4324) ccw projected
  arc A400 (50.2924, 30.3683) -> (49.8906, 31.024) centre (0, 0) ccw projected
  arc A401 (49.8906, 31.024) -> (51.3753, 32.8874) centre (39.318, 40.9704) ccw projected
  arc A402 (51.3753, 32.8874) -> (50.9404, 33.5571) centre (0, 0) ccw projected
  arc A403 (50.9404, 33.5571) -> (48.6342, 32.9588) centre (53.4204, 19.2546) ccw projected
  arc A404 (48.6342, 32.9588) -> (48.1986, 33.5925) centre (0, 0) ccw projected
  arc A405 (48.1986, 33.5925) -> (49.5836, 35.5311) centre (37.1199, 42.972) ccw projected
  arc A406 (49.5836, 35.5311) -> (49.1143, 36.1771) centre (0, 0) ccw projected
  arc A407 (49.1143, 36.1771) -> (46.8426, 35.4589) centre (52.3395, 22.0241) ccw projected
  arc A408 (46.8426, 35.4589) -> (46.3744, 36.069) centre (0, 0) ccw projected
  arc A409 (46.3744, 36.069) -> (47.6561, 38.0775) centre (34.8201, 44.8558) ccw projected
  arc A410 (47.6561, 38.0775) -> (47.1536, 38.698) centre (0, 0) ccw projected
  arc A411 (47.1536, 38.698) -> (44.9226, 37.8619) centre (51.1151, 24.7331) ccw projected
  arc A412 (44.9226, 37.8619) -> (44.4232, 38.4466) centre (0, 0) ccw projected
  arc A413 (44.4232, 38.4466) -> (45.598, 40.5194) centre (32.4248, 46.6167) ccw projected
  arc A414 (45.598, 40.5194) -> (45.0637, 41.1128) centre (0, 0) ccw projected
  arc A415 (45.0637, 41.1128) -> (42.8795, 40.161) centre (49.7506, 27.3744) ccw projected
  arc A416 (42.8795, 40.161) -> (42.3501, 40.7189) centre (0, 0) ccw projected
  arc A417 (42.3501, 40.7189) -> (43.4149, 42.8503) centre (29.9406, 48.2498) ccw projected
  arc A418 (43.4149, 42.8503) -> (42.8503, 43.4149) centre (0, 0) ccw projected
  arc A419 (42.8503, 43.4149) -> (40.7189, 42.3501) centre (48.2498, 29.9406) ccw projected
  arc A420 (40.7189, 42.3501) -> (40.161, 42.8795) centre (0, 0) ccw projected
  arc A421 (40.161, 42.8795) -> (41.1128, 45.0637) centre (27.3744, 49.7506) ccw projected
  arc A422 (41.1128, 45.0637) -> (40.5194, 45.598) centre (0, 0) ccw projected
  arc A423 (40.5194, 45.598) -> (38.4466, 44.4232) centre (46.6167, 32.4248) ccw projected
  arc A424 (38.4466, 44.4232) -> (37.8619, 44.9226) centre (0, 0) ccw projected
  arc A425 (37.8619, 44.9226) -> (38.698, 47.1536) centre (24.7331, 51.1151) ccw projected
  arc A426 (38.698, 47.1536) -> (38.0775, 47.6561) centre (0, 0) ccw projected
  arc A427 (38.0775, 47.6561) -> (36.069, 46.3744) centre (44.8558, 34.8201) ccw projected
  arc A428 (36.069, 46.3744) -> (35.4589, 46.8426) centre (0, 0) ccw projected
  arc A429 (35.4589, 46.8426) -> (36.1771, 49.1143) centre (22.0241, 52.3395) ccw projected
  arc A430 (36.1771, 49.1143) -> (35.5311, 49.5836) centre (0, 0) ccw projected
  arc A431 (35.5311, 49.5836) -> (33.5925, 48.1986) centre (42.972, 37.1199) ccw projected
  arc A432 (33.5925, 48.1986) -> (32.9588, 48.6342) centre (0, 0) ccw projected
  arc A433 (32.9588, 48.6342) -> (33.5571, 50.9404) centre (19.2546, 53.4204) ccw projected
  arc A434 (33.5571, 50.9404) -> (32.8874, 51.3753) centre (0, 0) ccw projected
  arc A435 (32.8874, 51.3753) -> (31.024, 49.8906) centre (40.9704, 39.318) ccw projected
  arc A436 (31.024, 49.8906) -> (30.3683, 50.2924) centre (0, 0) ccw projected
  arc A437 (30.3683, 50.2924) -> (30.8451, 52.6268) centre (16.4324, 54.3549) ccw projected
  arc A438 (30.8451, 52.6268) -> (30.1536, 53.026) centre (0, 0) ccw projected
  arc A439 (30.1536, 53.026) -> (28.3704, 51.4459) centre (38.8565, 41.4084) ccw projected
  arc A440 (28.3704, 51.4459) -> (27.6946, 51.8129) centre (0, 0) ccw projected
  arc A441 (27.6946, 51.8129) -> (28.0486, 54.169) centre (13.5652, 55.1404) ccw projected
  arc A442 (28.0486, 54.169) -> (27.3371, 54.5315) centre (0, 0) ccw projected
  arc A443 (27.3371, 54.5315) -> (25.639, 52.8602) centre (36.6361, 43.3852) ccw projected
  arc A444 (25.639, 52.8602) -> (24.9449, 53.1913) centre (0, 0) ccw projected
  arc A445 (24.9449, 53.1913) -> (25.1751, 55.5627) centre (10.6608, 55.7748) ccw projected
  arc A446 (25.1751, 55.5627) -> (24.4457, 55.8875) centre (0, 0) ccw projected
  arc A447 (24.4457, 55.8875) -> (22.8374, 54.1296) centre (34.3153, 45.2431) ccw projected
  arc A448 (22.8374, 54.1296) -> (22.1269, 54.4239) centre (0, 0) ccw projected
  arc A449 (22.1269, 54.4239) -> (22.2327, 56.8041) centre (7.7272, 56.2563) ccw projected
  arc A450 (22.2327, 56.8041) -> (21.4873, 57.0903) centre (0, 0) ccw projected
  arc A451 (21.4873, 57.0903) -> (19.9732, 55.2506) centre (31.9004, 46.977) ccw projected
  arc A452 (19.9732, 55.2506) -> (19.2483, 55.5074) centre (0, 0) ccw projected
  arc A453 (19.2483, 55.5074) -> (19.2293, 57.8898) centre (4.7723, 56.5836) ccw projected
  arc A454 (19.2293, 57.8898) -> (18.4699, 58.1366) centre (0, 0) ccw projected
  arc A455 (18.4699, 58.1366) -> (17.0542, 56.2202) centre (29.3981, 48.5822) ccw projected
  arc A456 (17.0542, 56.2202) -> (16.3169, 56.4387) centre (0, 0) ccw projected
  arc A457 (16.3169, 56.4387) -> (16.1733, 58.8169) centre (1.8044, 56.7558) ccw projected
  arc A458 (16.1733, 58.8169) -> (15.402, 59.0235) centre (0, 0) ccw projected
  arc A459 (15.402, 59.0235) -> (14.0885, 57.0357) centre (26.8152, 50.0542) ccw projected
  arc A460 (14.0885, 57.0357) -> (13.3407, 57.2153) centre (0, 0) ccw projected
  arc A461 (13.3407, 57.2153) -> (13.0729, 59.5827) centre (-1.1684, 56.7725) ccw projected
  arc A462 (13.0729, 59.5827) -> (12.2918, 59.7487) centre (0, 0) ccw projected
  arc A463 (12.2918, 59.7487) -> (11.0842, 57.6949) centre (24.1588, 51.389) ccw projected
  arc A464 (11.0842, 57.6949) -> (10.328, 57.8351) centre (0, 0) ccw projected
  arc A465 (10.328, 57.8351) -> (9.9366, 60.1852) centre (-4.138, 56.6335) ccw projected
  arc A466 (9.9366, 60.1852) -> (9.148, 60.3102) centre (0, 0) ccw projected
  arc A467 (9.148, 60.3102) -> (8.0495, 58.1959) centre (21.4362, 52.5829) ccw projected
  arc A468 (8.0495, 58.1959) -> (7.287, 58.2963) centre (0, 0) ccw projected
  arc A469 (7.287, 58.2963) -> (6.7732, 60.6228) centre (-7.0963, 56.3393) ccw projected
  arc A470 (6.7732, 60.6228) -> (5.979, 60.7063) centre (0, 0) ccw projected
  arc A471 (5.979, 60.7063) -> (4.9927, 58.5375) centre (18.6549, 53.6328) ccw projected
  arc A472 (4.9927, 58.5375) -> (4.226, 58.5978) centre (0, 0) ccw projected
  arc A473 (4.226, 58.5978) -> (3.5911, 60.8942) centre (-10.0352, 55.8907) ccw projected
  arc A474 (3.5911, 60.8942) -> (2.7937, 60.936) centre (0, 0) ccw projected
  arc A475 (2.7937, 60.936) -> (1.9222, 58.7185) centre (15.8224, 54.5356) ccw projected
  arc A476 (1.9222, 58.7185) -> (1.1535, 58.7387) centre (0, 0) ccw projected
  arc A477 (1.1535, 58.7387) -> (0.3992, 60.9987) centre (-12.9465, 55.2889) ccw projected
  arc A478 (0.3992, 60.9987) -> (-0.3992, 60.9987) centre (0, 0) ccw projected
  arc A479 (-0.3992, 60.9987) -> (-1.1535, 58.7387) centre (12.9465, 55.2889) ccw projected
  arc A480 (-1.1535, 58.7387) -> (-1.9222, 58.7185) centre (0, 0) ccw projected
  arc A481 (-1.9222, 58.7185) -> (-2.7937, 60.936) centre (-15.8224, 54.5356) ccw projected
  arc A482 (-2.7937, 60.936) -> (-3.5911, 60.8942) centre (0, 0) ccw projected
equation "\"d0\" = da_da"
equation "\"d1\" = da_b"
equation "\"d3\" = da_d"
equation "\"d16\" = da_aw"
equation "\"d43\" = da_aw"
equation "\"d46\" = da_aw"
equation "\"da_da\" = 122"
equation "\"da_b\" = 6"
equation "\"da_d\" = 120"
equation "\"da_aw\" = 76"
body "Solid1"
body "Srf1"
